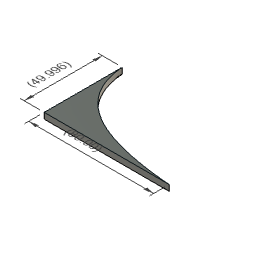
ramp (Autodesk Fusion 360 design; units mm, degrees)
Autodesk Fusion 360 part; units mm, degrees
sketch "Sketch1" plane through (0, 0, 0) normal (0, 0, 1) x (1, 0, 0)
  line L0 (0, 0) -> (80, 0)
  line L1 (80, 0) -> (80, 80) construction
  line L2 (80, 80) -> (0, 80) construction
  line L3 (0, 80) -> (0, 0)
  spline S0 degree 5 poles (80, 0) (79.8453, 0) (78.9706, 0.0526) (75.9629, 0.2894) (68.8602, 0.9688) (56.4676, 2.7021) (42.5797, 5.6691) (29.177, 10.2076) (17.7231, 16.518) (8.8897, 24.5903) (2.9106, 34.3304) (0.3908, 43.3608) (-0.2734, 50.789) (-0.1804, 56.0276) (0, 58.7185) knots 0 0 0 0 0 0 0.1 0.2 0.3 0.4 0.5 0.6 0.7 0.8 0.9 1 1 1 1 1 1
  line L4 (80.8669, 0) -> (79.1331, 0)
  point P0 (32.9492, 9.2849)
  constraint coincident L0.start L3.end
  constraint horizontal L0
  constraint perpendicular L0 L1
  constraint perpendicular L1 L2
  constraint perpendicular L0 L3
  constraint coincident L3 S0.end
  constraint midpoint L0.end L4
  constraint coincident L0 L4.end
extrude "Extrude1" add sketch "Sketch1" along normal blind 3.8 contours L0 L3 S0 L4
sketch "Sketch2" plane through (0, 0, 3.8) normal (0, 0, 1) x (-1, 0, 0)
  spline S0 degree 5 poles (-80, 0) (-79.8453, 0) (-78.9706, -0.0526) (-75.9629, -0.2894) (-68.8602, -0.9688) (-56.4676, -2.7021) (-42.5797, -5.6691) (-29.177, -10.2076) (-17.7231, -16.518) (-8.8897, -24.5903) (-3.7147, -33.0206) (-1.3019, -40.3599) (-0.3584, -45.8937) (-0.0593, -49.1781) (0, -49.9963) knots 0 0 0 0 0 0 0.1 0.2 0.3 0.4 0.5 0.6 0.7 0.8 0.9 0.932762 0.932762 0.932762 0.932762 0.932762 0.932762
  line L0 (0, -49.9963) -> (0, 0)
  line L1 (0, 0) -> (-80, 0)
  dimension "d3" = 80
  dimension "d4" = 49.9963
  measures "d3" distance of S0.start L0.end
  measures "d4" distance of S0.end L0.end
